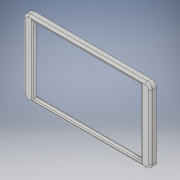
# Autodesk Inventor part: Touch screen front box part
Saved by Autodesk Inventor 2018 (Build 220112000, 112)
## iProperties
Created: 2019-09-12
Part Number: Touch screen front box part
Material: Generic
Document SubType Name: Modeling
Designer: Jacob
Density: 1 g/cm^3
Appearance: Default
Author: Jacob
Autodesk Inventor part; units mm, degrees
ref_plane "YZ Plane" through (0, 0, 0) normal (1, 0, 0) x (0, 1, 0)
ref_plane "XZ Plane" through (0, 0, 0) normal (0, 1, 0) x (-1, 0, 0)
ref_plane "XY Plane" through (0, 0, 0) normal (0, 0, 1) x (1, 0, 0)
sketch "Sketch1" plane through (0, 0, 0) normal (0, 0, 1) x (1, 0, 0)
  line L0 (-82.675, 50.375) -> (82.675, 50.375)
  line L1 (82.675, 50.375) -> (82.675, -50.375)
  line L2 (82.675, -50.375) -> (-82.675, -50.375)
  line L3 (-82.675, -50.375) -> (-82.675, 50.375)
  line L4 (-82.675, 50.375) -> (82.675, -50.375) construction
  line L5 (82.675, 50.375) -> (-82.675, -50.375) construction
  line L6 (-96.5, 55.5) -> (96.5, 55.5)
  line L7 (96.5, 55.5) -> (96.5, -55.5)
  line L8 (96.5, -55.5) -> (-96.5, -55.5)
  line L9 (-96.5, -55.5) -> (-96.5, 55.5)
  line L10 (-96.5, 55.5) -> (96.5, -55.5) construction
  line L11 (96.5, 55.5) -> (-96.5, -55.5) construction
  point P0 (0, 0)
  dimension "d0" = 165.35
  dimension "d1" = 100.75
  dimension "d2" = 111
  dimension "d3" = 193
  constraints: 24 end point, 4 midpoint, 4 parallel, 2 horizontal, 2 perpendicular
  measures "d0" distance of L0.start L0.end
  measures "d1" distance of L0.end L1.end
  measures "d2" distance of L8.end L6.start
  measures "d3" distance of L7.end L8.end
extrude "Extrusion1" add sketch "Sketch1" along normal blind 3.175
sketch "Sketch2" plane through (0, 0, 3.175) normal (0, 0, 1) x (1, 0, 0)
  line L0 (-99.675, 58.675) -> (99.675, 58.675)
  line L1 (99.675, 58.675) -> (99.675, -58.675)
  line L2 (99.675, -58.675) -> (-99.675, -58.675)
  line L3 (-99.675, -58.675) -> (-99.675, 58.675)
  line L4 (-99.675, 58.675) -> (99.675, -58.675) construction
  line L5 (99.675, 58.675) -> (-99.675, -58.675) construction
  line L6 (96.5, 55.5) -> (-96.5, 55.5) projected
  line L7 (96.5, -55.5) -> (96.5, 55.5) projected
  line L8 (82.675, -50.375) -> (82.675, 50.375) projected
  line L9 (-82.675, 50.375) -> (82.675, 50.375)
  line L10 (82.675, 50.375) -> (82.675, -50.375)
  line L11 (82.675, -50.375) -> (-82.675, -50.375)
  line L12 (-82.675, -50.375) -> (-82.675, 50.375)
  line L13 (-82.675, 50.375) -> (82.675, -50.375) construction
  line L14 (82.675, 50.375) -> (-82.675, -50.375) construction
  point P0 (0, 0)
  point P1 (88.5, 55.5)
  point P2 (-88.5, 55.5)
  point P3 (96.5, -47.5)
  point P4 (96.5, 47.5)
  dimension "d7" = 3.175
  dimension "d8" = 3.175
  constraints: 24 end point, 4 midpoint, 4 parallel, 2 horizontal, 2 perpendicular
  measures "d7" distance between parallel lines of L0 L6
  measures "d8" distance between parallel lines of L7 L1
extrude "Extrusion2" add sketch "Sketch2" against normal blind 3.175
fillet "Fillet2" radius 8 4 edges at (99.675, 58.675, 1.5875) (99.675, -58.675, 1.5875) (-99.675, -58.675, 1.5875) (-99.675, 58.675, 1.5875)
sketch "Sketch3" plane through (0, 0, 0) normal (0, 0, -1) x (-1, 0, 0)
  line L0 (-88.5, 55.5) -> (88.5, 55.5)
  line L1 (96.5, 47.5) -> (96.5, -47.5)
  line L2 (88.5, -55.5) -> (-88.5, -55.5)
  line L3 (-96.5, -47.5) -> (-96.5, 47.5)
  line L4 (-96.5, 55.5) -> (96.5, -55.5) construction
  line L5 (96.5, 55.5) -> (-96.5, -55.5) construction
  line L6 (91.675, 58.675) -> (-91.675, 58.675) projected
  line L7 (99.675, -50.675) -> (99.675, 50.675) projected
  arc A0 (-88.5, 55.5) -> (-96.5, 47.5) centre (-88.5, 47.5) ccw
  arc A1 (96.5, 47.5) -> (88.5, 55.5) centre (88.5, 47.5) ccw
  arc A2 (88.5, -55.5) -> (96.5, -47.5) centre (88.5, -47.5) ccw
  arc A3 (-96.5, -47.5) -> (-88.5, -55.5) centre (-88.5, -47.5) ccw
  line L8 (-91.675, 58.675) -> (91.675, 58.675)
  line L9 (99.675, 50.675) -> (99.675, -50.675)
  line L10 (91.675, -58.675) -> (-91.675, -58.675)
  line L11 (-99.675, -50.675) -> (-99.675, 50.675)
  line L12 (-99.675, 58.675) -> (99.675, -58.675) construction
  line L13 (99.675, 58.675) -> (-99.675, -58.675) construction
  arc A4 (-91.675, 58.675) -> (-99.675, 50.675) centre (-91.675, 50.675) ccw
  arc A5 (99.675, 50.675) -> (91.675, 58.675) centre (91.675, 50.675) ccw
  arc A6 (91.675, -58.675) -> (99.675, -50.675) centre (91.675, -50.675) ccw
  arc A7 (-99.675, -50.675) -> (-91.675, -58.675) centre (-91.675, -50.675) ccw
  point P0 (0, 0)
  dimension "d12" = 3.175
  dimension "d13" = 3.175
  dimension "d14" = 8
  dimension "d15" = 8
  constraints: 24 end point, 16 point on circle, 16 point on line, 16 tangent, 8 centre point, 6 equal radius, 4 midpoint, 4 parallel, 2 horizontal, 2 perpendicular
  measures "d12" distance between parallel lines of L6 L0
  measures "d13" distance between parallel lines of L7 L1
  measures "d14" radius of A0
  measures "d15" radius of A4
extrude "Extrusion3" add sketch "Sketch3" along normal blind 6.35
fillet "Fillet3" radius 3.175 8 edges at (97.3319, 56.3319, 3.175) (99.675, 0, 3.175) (97.3319, -56.3319, 3.175) (0, -58.675, 3.175) (-97.3319, -56.3319, 3.175) (-99.675, 0, 3.175) (-97.3319, 56.3319, 3.175) (0, 58.675, 3.175)
chamfer "Chamfer1" distance 3.175 angle 45 4 edges at (0, 50.375, 3.175) (-82.675, 0, 3.175) (82.675, 0, 3.175) (0, -50.375, 3.175)
fillet "Fillet4" radius 3.175 4 edges at (-85.8499, 0, 3.175) (0, 53.5499, 3.175) (85.8499, 0, 3.175) (0, -53.5499, 3.175)
sketch "Sketch4" plane through (0, 0, -6.35) normal (0, 0, -1) x (-1, 0, 0)
  arc A0 (-88.5, 55.5) -> (-96.5, 47.5) centre (-88.5, 47.5) ccw projected
  arc A1 (-91.675, 58.675) -> (-99.675, 50.675) centre (-91.675, 50.675) ccw projected
  line L0 (88.5, 55.5) -> (-88.5, 55.5) projected
  line L1 (-88.5, 55.5) -> (-96.5, 55.5) construction
  line L2 (-96.5, 47.5) -> (-96.5, 55.5) construction
  line L3 (-96.5, 50.675) -> (-96.5, -50.675) projected
  line L4 (-94.1569, 53.1569) -> (-97.3319, 56.3319) construction
  circle A2 centre (-95.7444, 54.7444) radius 0.7937
  arc A3 (96.5, 47.5) -> (88.5, 55.5) centre (88.5, 47.5) ccw projected
  line L5 (96.5, 47.5) -> (96.5, 55.5) construction
  line L6 (88.5, 55.5) -> (96.5, 55.5) construction
  line L7 (91.675, 55.5) -> (-91.675, 55.5) projected
  line L8 (94.1569, 53.1569) -> (97.3319, 56.3319) construction
  arc A4 (99.675, 50.675) -> (91.675, 58.675) centre (91.675, 50.675) ccw projected
  circle A5 centre (95.7444, 54.7444) radius 0.7937
  line L9 (-91.675, -55.5) -> (91.675, -55.5) projected
  line L10 (88.5, -55.5) -> (96.5, -55.5) construction
  line L11 (96.5, -55.5) -> (96.5, -47.8482) construction
  line L12 (96.5, -50.675) -> (96.5, 50.675) projected
  arc A6 (88.5, -55.5) -> (96.5, -47.5) centre (88.5, -47.5) ccw projected
  line L13 (97.3319, -56.3319) -> (94.1569, -53.1569) construction
  circle A7 centre (95.7444, -54.7444) radius 0.7937
  arc A8 (-96.5, -47.5) -> (-88.5, -55.5) centre (-88.5, -47.5) ccw projected
  line L14 (-88.5, -55.5) -> (-96.5, -55.5) construction
  arc A9 (-96.5, -50.675) -> (-91.675, -55.5) centre (-91.675, -50.675) ccw projected
  line L15 (-96.5, -55.5) -> (-96.5, -50.675) construction
  line L16 (-94.1569, -53.1569) -> (-97.3319, -56.3319) construction
  arc A10 (-99.675, -50.675) -> (-91.675, -58.675) centre (-91.675, -50.675) ccw projected
  circle A11 centre (-95.7444, -54.7444) radius 0.7937
  line L17 (91.675, 58.675) -> (-91.675, 58.675) projected
  line L18 (0, 58.675) -> (0, 55.5) construction
  circle A12 centre (0, 57.0875) radius 0.7937
  line L19 (0, -55.5) -> (0, -58.675) construction
  circle A13 centre (0, -57.0875) radius 0.7937
  line L20 (96.5, 0) -> (99.675, 0) construction
  circle A14 centre (98.0875, 0) radius 0.7937
  line L21 (-99.675, 50.675) -> (-99.675, -50.675) projected
  line L22 (-99.675, 0) -> (-96.5, 0) construction
  circle A15 centre (-98.0875, 0) radius 0.7937
  point P0 (0, 0)
  dimension "d25" = 1.5875
  dimension "d26" = 1.5875
  dimension "d27" = 1.5875
  dimension "d28" = 1.5875
  dimension "d29" = 1.5875
  dimension "d30" = 1.5875
  dimension "d31" = 1.5875
  dimension "d32" = 1.5875
  constraints: 32 end point, 14 midpoint, 8 centre point, 7 point on circle, 4 point on line, 4 tangent, 2 collinear, 1 horizontal, 1 perpendicular, 1 vertical
  measures "d25" diameter of A2
  measures "d26" diameter of A5
  measures "d27" diameter of A7
  measures "d28" diameter of A11
  measures "d29" diameter of A12
  measures "d30" diameter of A13
  measures "d31" diameter of A14
  measures "d32" diameter of A15
extrude "Extrusion4" cut sketch "Sketch4" against normal blind 6.35 contours A2 | A5 | A7 | A11 | A12 | A13 | A14 | A15
body "Solid1"
